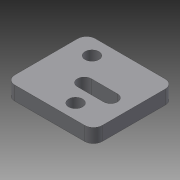
# Autodesk Inventor part: Carriage_Joint_Beltflap
Saved by Autodesk Inventor 2014 (Build 180170000, 170)
## iProperties
Created: 2014-10-17
Part Number: Carriage_Joint_Beltflap
Material: Generic
Document SubType Name: Modeling
Designer: ThatOtherGuy
Density: 1 g/cm^3
Appearance: Default
Author: ThatOtherGuy
Autodesk Inventor part; units mm, degrees
ref_plane "YZ Plane" through (0, 0, 0) normal (1, 0, 0) x (0, 1, 0)
ref_plane "XZ Plane" through (0, 0, 0) normal (0, 1, 0) x (-1, 0, 0)
ref_plane "XY Plane" through (0, 0, 0) normal (0, 0, 1) x (1, 0, 0)
sketch "Sketch1" plane through (0, 0, 0) normal (0, 0, 1) x (1, 0, 0)
  circle A0 centre (0, 0) radius 1.59
  line L0 (-12.5, 15) -> (7.5, 15)
  line L1 (7.5, 15) -> (7.5, -15)
  line L2 (7.5, -15) -> (-12.5, -15)
  line L3 (-12.5, -15) -> (-12.5, 15)
  circle A1 centre (-7.5, 11.25) radius 1.59
  line L4 (-3, 5) -> (3, 5) construction
  line L5 (-3, 3.4125) -> (3, 3.4125)
  line L6 (3, 6.5875) -> (-3, 6.5875)
  arc A2 (-3, 6.5875) -> (-3, 3.4125) centre (-3, 5) ccw
  arc A3 (3, 3.4125) -> (3, 6.5875) centre (3, 5) ccw
  line L7 (-3, -5) -> (3, -5) construction
  line L8 (-3, -6.5875) -> (3, -6.5875)
  line L9 (3, -3.4125) -> (-3, -3.4125)
  arc A4 (-3, -3.4125) -> (-3, -6.5875) centre (-3, -5) ccw
  arc A5 (3, -6.5875) -> (3, -3.4125) centre (3, -5) ccw
  line L10 (-12.5, -3.4125) -> (7.5, -3.4125)
  point P0 (7.5, 0)
  point P1 (0, 5)
  point P2 (0, -5)
  point P3 (0, 0)
  dimension "d2" = 3.18
  dimension "d31" = 20
  dimension "d32" = 30
  dimension "d33" = 10
  dimension "d35" = 5
  dimension "d39" = 3.175
  dimension "d41" = 6
  dimension "d42" = 9.175
  dimension "d44" = 7.5
  dimension "d45" = 15
  dimension "d46" = 11.25
  constraints: 26 end point, 8 point on circle, 8 tangent, 6 centre point, 6 parallel, 3 midpoint, 3 point on line, 2 equal radius, 2 horizontal, 2 perpendicular, 2 vertical alignment, 1 coincident, 1 horizontal alignment
  measures "d2" diameter of A0
  measures "d31" distance of L0.start L0.end
  measures "d32" distance of L2.end L0.start
  measures "d33" distance between parallel lines of L7 L4
  measures "d35" distance from line of point (0, 0) L4
  measures "d39" distance between parallel lines of L5 L6
  measures "d41" distance of L4.start L4.end
  measures "d44" distance from line of L1 A0.centre
  measures "d45" distance from line of L1 A1.centre
  measures "d46" vertical distance of A0.centre A1.centre
extrude "Extrusion1" add sketch "Sketch1" along normal blind 3.175 contours L0 L1 L10 L9 L3
fillet "Fillet1" radius 2 4 edges at (-12.5, 15, 1.5875) (7.5, 15, 1.5875) (7.5, -3.4125, 1.5875) (-12.5, -3.4125, 1.5875)
equation "\"d35\" = 0.5 * d33"
equation "\"d12\" = THICKA"
equation "\"THICKA\" = 3.175"
equation "\"THICKB\" = 6.731"
equation "\"THICKC\" = 12.7"
equation "\"MAGDIA\" = 9.5"
equation "\"BALLDIA\" = 12"
equation "\"THICKPLY\" = 5"
body "Solid1"
